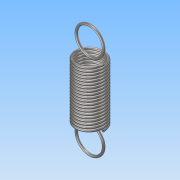
# Autodesk Inventor part: Spring_Extension
Saved by Autodesk Inventor 2017.3 (Build 213256000, 256)
## iProperties
Created: 2019-06-23
Part Number: Spring_Extension
Material: Steel, Carbon
Document SubType Name: Modeling
Designer: Derek Wider
Density: 7.85 g/cm^3
Appearance: Semi-Polished
Author: Derek Wider
Autodesk Inventor part; units mm, degrees
ref_plane "YZ Plane" through (0, 0, 0) normal (1, 0, 0) x (0, 1, 0)
ref_plane "XZ Plane" through (0, 0, 0) normal (0, 1, 0) x (-1, 0, 0)
ref_plane "XY Plane" through (0, 0, 0) normal (0, 0, 1) x (1, 0, 0)
sketch "Sketch1" plane through (0, 0, 0) normal (0, 0, 1) x (1, 0, 0)
  line L0 (0, 0) -> (0, 5.6417) construction
  circle A0 centre (2.413, 0) radius 0.235
  dimension "d0" = 2.413
  dimension "d1" = 0.4699
  constraints: 2 end point, 1 centre point, 1 vertical
  measures "d0" distance from line of L0 A0.centre
  measures "d1" diameter of A0
coil "Coil1" sketch "Sketch1" operation add axis through (0, 0, 0) along (0, 1, 0) pitch 0.5334 turns 20 hand right
sketch "Sketch2" plane through (0, 0, 0) normal (1, 0, 0) x (0, 1, 0)
  circle A0 centre (0, 0) radius 0.2349
  line L0 (-2.54, 0) -> (-2.54, -1.583)
  line L1 (10.433, 0) -> (10.903, 0) construction
  circle A1 centre (10.668, 0) radius 0.2349
  line L2 (13.208, 0) -> (13.208, -1.7963) construction
  point P0 (0, 0)
  dimension "d10" = 0.4699
  dimension "d11" = 2.54
  dimension "d12" = 0.4699
  dimension "d13" = 2.54
  constraints: 4 end point, 2 centre point, 2 coincident, 2 vertical
  measures "d10" diameter of A0
  measures "d11" distance from line of point (0, 0) L0
  measures "d12" diameter of A1
  measures "d13" distance from line of A1.centre L2
revolve "Revolution1" add sketch "Sketch2" angle 360 about axis through (0, 13.208, 0) along (0, 0, -1) contours A1
revolve "Revolution2" add sketch "Sketch2" angle 360 about axis through (0, -2.54, 0) along (0, 0, -1) contours A0
body "Solid1"
